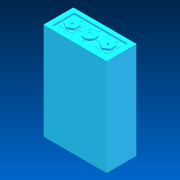
# Autodesk Inventor part: CALB100AH final
Saved by Autodesk Inventor 2012 (Build 160160000, 160)
## iProperties
Created: 2012-07-03
Part Number: CALB100AH final
Material: Default
Document SubType Name: Sheet Metal
Designer: Hemant
Density: 1 g/cm^3
Sheet Metal Rule: Default
Author: Hemant
Autodesk Inventor part; units mm, degrees
ref_plane "YZ Plane" through (0, 0, 0) normal (1, 0, 0) x (0, 1, 0)
ref_plane "XZ Plane" through (0, 0, 0) normal (0, 1, 0) x (-1, 0, 0)
ref_plane "XY Plane" through (0, 0, 0) normal (0, 0, 1) x (1, 0, 0)
sketch "Sketch1" plane through (0, 0, 0) normal (0, 0, 1) x (1, 0, 0)
  line L0 (0, 0) -> (-142, 0)
  line L1 (-142, 0) -> (-142, 218)
  line L2 (-142, 218) -> (0, 218)
  line L3 (0, 218) -> (0, 0)
  dimension "d0" = 142
  dimension "d1" = 218
  constraints: 8 end point, 2 parallel, 1 horizontal, 1 perpendicular
  measures "d0" distance of L1.end L2.end
  measures "d1" distance of L0.end L1.end
extrude "Extrusion1" add sketch "Sketch1" along normal blind 67
sketch "Sketch6" plane through (-142, 218, 0) normal (0, 1, 0) x (1, 0, 0)
  line L0 (0, -67) -> (142, -67) projected
  line L1 (142, 0) -> (142, -67) projected
  line L2 (0, 0) -> (142, 0) projected
  line L3 (0, 0) -> (0, -67) projected
  line L4 (11, -9) -> (131, -9)
  line L5 (131, -9) -> (131, -58)
  line L6 (131, -58) -> (11, -58)
  line L7 (11, -58) -> (11, -9)
  dimension "d33" = 67
  dimension "d34" = 142
  dimension "d35" = 11
  dimension "d36" = 11
  dimension "d37" = 9
  dimension "d38" = 9
  constraints: 8 end point, 2 parallel, 1 horizontal, 1 perpendicular
  measures "d33" distance between parallel lines of L0 L2
  measures "d34" distance between parallel lines of L1 L3
  measures "d35" distance between parallel lines of L3 L7
  measures "d36" distance between parallel lines of L1 L5
  measures "d37" distance between parallel lines of L0 L6
  measures "d38" distance between parallel lines of L2 L4
extrude "Extrusion5" cut sketch "Sketch6" against normal blind 4 contours L4 L5 L6 L7
sketch "Sketch7" plane through (-142, 214, 0) normal (0, 1, 0) x (1, 0, 0)
  line L0 (11, -58) -> (131, -58) projected
  line L1 (131, -58) -> (131, -9) projected
  line L2 (11, -9) -> (131, -9)
  line L3 (131, -9) -> (131, -58)
  line L4 (131, -58) -> (11, -58)
  line L5 (11, -58) -> (11, -9)
  line L6 (11, -9) -> (11, -32)
  line L7 (11, -32) -> (11, -35)
  line L8 (11, -35) -> (11, -58)
  line L9 (11, -32) -> (16, -32)
  line L10 (11, -35) -> (16, -35)
  line L11 (11, -9) -> (29, -9)
  line L12 (29, -9) -> (32, -9)
  line L13 (32, -9) -> (69.5, -9)
  line L14 (69.5, -9) -> (72.5, -9)
  line L15 (72.5, -9) -> (110, -9)
  line L16 (131, -9) -> (113, -9)
  line L17 (113, -9) -> (110, -9)
  line L18 (29, -9) -> (29, -18.5)
  line L19 (32, -18.5) -> (32, -9)
  line L20 (29, -9) -> (32, -9)
  line L21 (32, -58) -> (32, -48.5)
  line L22 (29, -48.5) -> (29, -58)
  line L23 (16, -48.5) -> (16, -35)
  line L24 (16, -32) -> (16, -18.5)
  line L25 (16, -18.5) -> (29, -18.5)
  line L26 (32, -18.5) -> (46, -18.5)
  line L27 (46, -18.5) -> (46, -32)
  line L28 (46, -35) -> (46, -48.5)
  line L29 (69.5, -9) -> (69.5, -32)
  line L30 (69.5, -35) -> (69.5, -58)
  line L31 (72.5, -9) -> (72.5, -32)
  line L32 (72.5, -35) -> (72.5, -58)
  line L33 (46, -32) -> (69.5, -32)
  line L34 (46, -35) -> (69.5, -35)
  line L35 (72.5, -35) -> (96, -35)
  line L36 (126, -35) -> (131, -35)
  line L37 (110, -9) -> (110, -18.5)
  line L38 (110, -48.5) -> (110, -58)
  line L39 (72.5, -32) -> (96, -32)
  line L40 (126, -32) -> (131, -32)
  line L41 (113, -9) -> (113, -18.5)
  line L42 (110, -58) -> (110, -48.5)
  line L43 (110, -18.5) -> (110, -9)
  line L44 (113, -48.5) -> (113, -58)
  line L45 (126, -48.5) -> (113, -48.5)
  line L46 (110, -48.5) -> (96, -48.5)
  line L47 (126, -18.5) -> (126, -32)
  line L48 (126, -35) -> (126, -48.5)
  line L49 (96, -48.5) -> (96, -35)
  line L50 (96, -32) -> (96, -18.5)
  line L51 (96, -18.5) -> (110, -18.5)
  line L52 (113, -18.5) -> (126, -18.5)
  line L53 (46, -48.5) -> (32, -48.5)
  line L54 (29, -48.5) -> (16, -48.5)
  line L55 (11, -32) -> (16, -32)
  line L56 (16, -18.5) -> (29, -18.5)
  line L57 (29, -9) -> (32, -9)
  line L58 (32, -18.5) -> (46, -18.5)
  line L59 (46, -32) -> (69.5, -32)
  line L60 (69.5, -9) -> (72.5, -9)
  line L61 (72.5, -32) -> (96, -32)
  line L62 (96, -18.5) -> (110, -18.5)
  line L63 (110, -9) -> (113, -9)
  line L64 (113, -18.5) -> (126, -18.5)
  line L65 (126, -32) -> (131, -32)
  line L66 (131, -35) -> (126, -35)
  line L67 (126, -48.5) -> (113, -48.5)
  line L68 (113, -58) -> (110, -58)
  line L69 (110, -48.5) -> (96, -48.5)
  line L70 (96, -35) -> (72.5, -35)
  line L71 (72.5, -58) -> (69.5, -58)
  line L72 (69.5, -35) -> (46, -35)
  line L73 (46, -48.5) -> (32, -48.5)
  line L74 (32, -58) -> (29, -58)
  line L75 (29, -48.5) -> (16, -48.5)
  line L76 (16, -35) -> (11, -35)
  point P0 (142, 0)
  constraints: 150 end point, 34 parallel, 33 perpendicular, 17 point on line, 11 collinear, 5 horizontal
extrude "Extrusion6" add sketch "Sketch7" along normal blind 1 contours L22 L54 L23 L10 L5 L9 L24 L25 L18 L2 L19 L26 L27 L33 L29 L31 L39 L50 L51 L37 L41 L52 L47 L40 L1 L36 L48 L45 L44 L0 L38 L46 L49 L35 L32 L30 L34 L28 L53 L21
sketch "Sketch8" plane through (-142, 215, 0) normal (0, 1, 0) x (1, 0, 0)
  line L0 (126, -18.5) -> (126, -32) projected
  line L1 (113, -18.5) -> (126, -18.5) projected
  line L2 (32, -18.5) -> (46, -18.5) projected
  line L3 (16, -32) -> (16, -18.5) projected
  line L4 (31, -47.3564) -> (19, -40.4282)
  line L5 (19, -40.4282) -> (19, -26.5718)
  line L6 (19, -26.5718) -> (31, -19.6436)
  line L7 (31, -19.6436) -> (43, -26.5718)
  line L8 (43, -26.5718) -> (43, -40.4282)
  line L9 (43, -40.4282) -> (31, -47.3564)
  line L10 (110.8321, -19.6446) -> (122.9152, -26.4269)
  line L11 (122.9152, -26.4269) -> (123.0831, -40.2823)
  line L12 (123.0831, -40.2823) -> (111.1679, -47.3554)
  line L13 (111.1679, -47.3554) -> (99.0848, -40.5731)
  line L14 (99.0848, -40.5731) -> (98.9169, -26.7177)
  line L15 (98.9169, -26.7177) -> (110.8321, -19.6446)
  circle A0 centre (111, -33.5) radius 3.75
  circle A1 centre (31, -33.5) radius 3.75
  circle A2 centre (71, -33.5) radius 14
  point P0 (142, 0)
  dimension "d62" = 15
  dimension "d63" = 15
  dimension "d64" = 15
  dimension "d65" = 15
  dimension "d66" = 12
  dimension "d67" = 12
  dimension "d69" = 7.5
  dimension "d70" = 7.5
  dimension "d71" = 28
  constraints: 24 end point, 5 coincident, 3 centre point, 26 other
  measures "d62" distance from line of L2 point (31, -33.5)
  measures "d63" distance from line of point (31, -33.5) L3
  measures "d64" distance from line of L1 point (111, -33.5)
  measures "d65" distance from line of L0 point (111, -33.5)
  measures "d66" distance from line of L6 point (31, -33.5)
  measures "d67" distance from line of L15 point (111, -33.5)
  measures "d69" diameter of A0
  measures "d70" diameter of A1
  measures "d71" diameter of A2
extrude "Extrusion7" add sketch "Sketch8" along normal blind 4 contours L4 L5 L6 L7 L8 L9 | L10 L11 L12 L13 L14 L15 | A0 | A1 | A2
sketch "Sketch9" plane through (-71, 219, 33.5) normal (0, 1, 0) x (1, 0, 0)
  circle A0 centre (0, 0) radius 14 projected
  circle A1 centre (0, 0) radius 12.5
  point P0 (71, 33.5)
  dimension "d74" = 25
  constraints: 1 centre point, 1 coincident
  measures "d74" diameter of A1
extrude "Extrusion8" cut sketch "Sketch9" against normal blind 0.5 contours A1
sketch "Sketch10" plane through (-71, 218.5, 33.5) normal (0, 1, 0) x (1, 0, 0)
  circle A0 centre (0, 0) radius 12.5 projected
  line L0 (0, 4.6188) -> (4, 2.3094)
  line L1 (4, 2.3094) -> (4, -2.3094)
  line L2 (4, -2.3094) -> (0, -4.6188)
  line L3 (0, -4.6188) -> (-4, -2.3094)
  line L4 (-4, -2.3094) -> (-4, 2.3094)
  line L5 (-4, 2.3094) -> (0, 4.6188)
  circle A1 centre (0, 0) radius 1.5
  point P0 (71, 33.5)
  dimension "d77" = 4
  dimension "d78" = 3
  constraints: 12 end point, 2 coincident, 1 centre point, 13 other
  measures "d77" distance from line of A0.centre L1
  measures "d78" diameter of A1
extrude "Extrusion9" cut sketch "Sketch10" against normal blind 1 contours L0 L1 L2 L3 L4 L5 | A1
sketch "Sketch11" plane through (-71, 217.5, 33.5) normal (0, 1, 0) x (1, 0, 0)
  circle A0 centre (0, 0) radius 1.5
  point P0 (71, 33.5)
  dimension "d81" = 3
  constraints: 1 centre point
  measures "d81" diameter of A0
extrude "Extrusion10" cut sketch "Sketch11" against normal blind 0.1
sketch "Sketch13" plane through (-142, 219, 0) normal (0, 1, 0) x (1, 0, 0)
  circle A0 centre (31, -33.5) radius 2.5
  point P0 (142, 0)
  dimension "d84" = 5
  constraints: 1 centre point
  measures "d84" diameter of A0
extrude "Extrusion11" cut sketch "Sketch13" against normal blind 8
sketch "Sketch14" plane through (-142, 219, 0) normal (0, 1, 0) x (1, 0, 0)
  circle A0 centre (111, -33.5) radius 2.5
  point P0 (142, 0)
  dimension "d87" = 5
  constraints: 1 centre point
  measures "d87" diameter of A0
extrude "Extrusion12" cut sketch "Sketch14" against normal blind 8
equation "\"BendRadius\" = Thickness"
equation "\"BendReliefWidth\" = Thickness"
equation "\"BendReliefDepth\" = 0.5 * Thickness"
equation "\"CornerReliefSize\" = 4 * Thickness"
equation "\"MinimumRemnant\" = 2 * Thickness"
equation "\"TransitionRadius\" = BendRadius"
equation "\"JacobiRadiusSize\" = Thickness"
equation "\"GapSize\" = Thickness"
equation "\"Thickness\" = 0.5"
body "Solid1"
